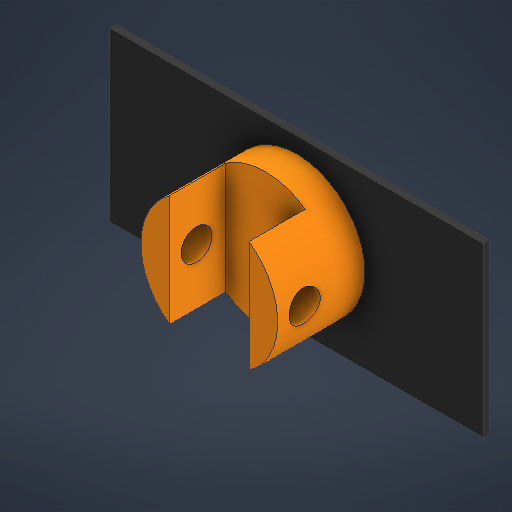
# Autodesk Inventor part: Proximal
Saved by Autodesk Inventor 2026 (Build 300175000, 175)
## iProperties
Created: 2026-01-04
Part Number: Proximal
Material: Generic
Document SubType Name: Modeling
Designer: saraswat22
Density: 1 g/cm^3
Appearance: Default
Author: saraswat22
Autodesk Inventor part; units mm, degrees
ref_plane "YZ Plane" through (0, 0, 0) normal (1, 0, 0) x (0, 1, 0)
ref_plane "XZ Plane" through (0, 0, 0) normal (0, 1, 0) x (-1, 0, 0)
ref_plane "XY Plane" through (0, 0, 0) normal (0, 0, 1) x (1, 0, 0)
sketch "Sketch3" plane through (0, 0, 0) normal (0, 0, 1) x (1, 0, 0)
  line L0 (-304.8, -137.16) -> (304.8, -137.16)
  line L1 (304.8, -137.16) -> (304.8, 137.16)
  line L2 (304.8, 137.16) -> (-304.8, 137.16)
  line L3 (-304.8, 137.16) -> (-304.8, -137.16)
  line L4 (-304.8, -137.16) -> (304.8, 137.16) construction
  line L5 (304.8, -137.16) -> (-304.8, 137.16) construction
  point P0 (0, 0)
  dimension "d0" = 609.6
  dimension "d1" = 274.32
  constraints: 12 end point, 2 midpoint, 2 parallel, 1 horizontal, 1 perpendicular
  measures "d0" distance of L1.end L2.end
  measures "d1" distance of L0.end L1.end
extrude "Extrusion1" add sketch "Sketch3" along normal blind 10.16
sketch "Sketch4" plane through (0, 0, 10.16) normal (0, 0, 1) x (1, 0, 0)
  circle A0 centre (0, 0) radius 111.76
  dimension "d4" = 223.52
  constraints: 1 centre point, 1 coincident
  measures "d4" diameter of A0
extrude "Extrusion2" add sketch "Sketch4" along normal blind 142.24
sketch "Sketch5" plane through (0, 0, 152.4) normal (0, 0, 1) x (1, 0, 0)
  line L0 (64.897, -91.9688) -> (64.897, 91.9688)
  line L1 (-64.897, 91.9688) -> (-64.897, -91.9688)
  line L2 (-64.897, -91.9688) -> (64.897, 91.9688) construction
  line L3 (64.897, -91.9688) -> (-64.897, 91.9688) construction
  arc A0 (-64.897, -91.9688) -> (64.897, -91.9688) centre (0, 4.5367) ccw
  arc A1 (64.897, 91.9688) -> (-64.897, 91.9688) centre (0, -4.5367) ccw
  point P0 (0, 0)
  constraints: 8 end point, 4 point on circle, 2 centre point, 2 midpoint, 1 parallel
extrude "Extrusion3" cut sketch "Sketch5" against normal blind 91.44
sketch "Sketch6" plane through (-64.897, -90.9872, 152.4) normal (1, 0, 0) x (0, 0, -1)
  circle A0 centre (44.0373, 90.9872) radius 25.4
  point P0 (152.4, 90.9872)
  dimension "d10" = 50.8
  constraints: 1 centre point
  measures "d10" diameter of A0
extrude "Extrusion4" cut sketch "Sketch6" against normal through all
sketch "Sketch7" plane through (64.897, -90.9872, 152.4) normal (-1, 0, 0) x (0, 0, 1)
  circle A0 centre (-44.0373, 90.9872) radius 25.4 projected
  circle A1 centre (-44.0373, 90.9872) radius 25.4
  point P0 (-152.4, 90.9872)
  constraints: 1 centre point, 1 coincident
extrude "Extrusion5" cut sketch "Sketch7" against normal through all
body "Solid1"
